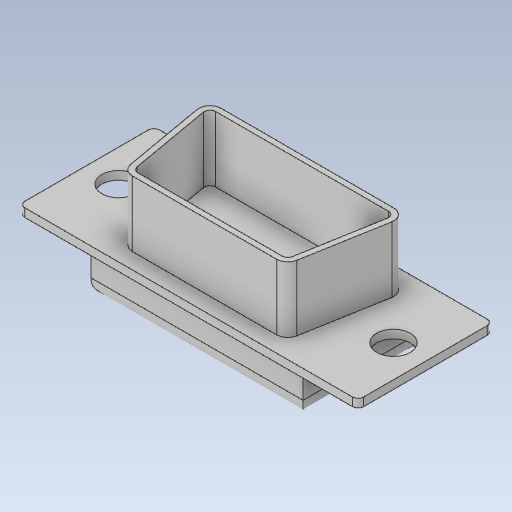
# Autodesk Inventor part: D-SUB
Saved by Autodesk Inventor 2020 (Build 240168000, 168)
## iProperties
Created: 2018-01-24
Part Number: D-SUB
Material: Generic
Document SubType Name: Modeling
Designer: Alex
Density: 1 g/cm^3
Appearance: Default
Author: Alex
Autodesk Inventor part; units mm, degrees
ref_plane "YZ Plane" through (0, 0, 0) normal (1, 0, 0) x (0, 1, 0)
ref_plane "XZ Plane" through (0, 0, 0) normal (0, 1, 0) x (-1, 0, 0)
ref_plane "XY Plane" through (0, 0, 0) normal (0, 0, 1) x (1, 0, 0)
sketch "Sketch1" plane through (0, 0, 0) normal (0, 1, 0) x (-1, 0, 0)
  line L0 (15.405, -6.125) -> (-15.405, -6.125)
  line L1 (-15.405, -6.125) -> (-15.405, 6.125)
  line L2 (-15.405, 6.125) -> (15.405, 6.125)
  line L3 (15.405, 6.125) -> (15.405, -6.125)
  line L4 (15.405, -6.125) -> (-15.405, 6.125) construction
  line L5 (-15.405, -6.125) -> (15.405, 6.125) construction
  point P0 (0, 0)
  point P1 (0, 0)
  dimension "d0" = 30.81
  dimension "d1" = 12.25
  constraints: 12 end point, 2 midpoint, 2 parallel, 1 coincident, 1 horizontal, 1 perpendicular
  measures "d0" distance of L1.end L2.end
  measures "d1" distance of L0.end L1.end
extrude "Extrusion1" add sketch "Sketch1" along normal blind 0.76
fillet "Fillet1" radius 0.5 4 edges at (15.405, 0.38, 6.125) (15.405, 0.38, -6.125) (-15.405, 0.38, 6.125) (-15.405, 0.38, -6.125)
sketch "Sketch2" plane through (0, 0.76, 0) normal (0, 1, 0) x (1, 0, 0)
  arc A0 (-14.905, 6.125) -> (-15.405, 5.625) centre (-14.905, 5.625) ccw construction
  line L0 (-15.405, 5.625) -> (-15.405, -5.625) construction
  arc A1 (-15.405, -5.625) -> (-14.905, -6.125) centre (-14.905, -5.625) ccw construction
  line L1 (-14.905, -6.125) -> (14.905, -6.125) construction
  arc A2 (14.905, -6.125) -> (15.405, -5.625) centre (14.905, -5.625) ccw construction
  line L2 (15.405, -5.625) -> (15.405, 5.625) construction
  arc A3 (15.405, 5.625) -> (14.905, 6.125) centre (14.905, 5.625) ccw construction
  line L3 (14.905, 6.125) -> (-14.905, 6.125) construction
  line L4 (-14.905, 6.125) -> (14.905, 6.125) construction
  line L5 (0, 6.125) -> (0, -6.125) construction
  line L6 (-14.905, -6.125) -> (14.905, -6.125) construction
  point P0 (0, 0)
  point P1 (-12.495, 0)
  point P2 (12.495, 0)
  point P3 (0, 0)
  dimension "d5" = 24.99
  constraints: 3 midpoint, 2 end point, 2 horizontal alignment, 1 symmetric about line
  measures "d5" distance of point (12.495, 0) point (-12.495, 0)
hole "Hole1" at (-12.495, 0.76, 0) at (12.495, 0.76, 0) direction (0, -1, 0) diameter 3.05 depth 8 tip angle 118
sketch "Sketch3" plane through (0, 0.76, 0) normal (0, 1, 0) x (1, 0, 0)
  line L0 (-7.8641, 4.18) -> (7.8641, 4.18)
  line L1 (8.3565, 3.5932) -> (7.0588, -3.7668)
  line L2 (6.5664, -4.18) -> (-6.5664, -4.18)
  line L3 (-7.0588, -3.7668) -> (-8.3565, 3.5932)
  line L4 (-14.905, 6.125) -> (14.905, 6.125) projected
  line L5 (0, 6.125) -> (0, -6.125) construction
  line L6 (-15.405, 0) -> (15.405, 0) construction
  line L7 (15.405, 5.625) -> (15.405, -5.625) projected
  circle A0 centre (-12.495, 0) radius 1.525 construction
  circle A1 centre (12.495, 0) radius 1.525 construction
  arc A2 (-14.905, 6.125) -> (-15.405, 5.625) centre (-14.905, 5.625) ccw construction
  line L8 (-15.405, 5.625) -> (-15.405, -5.625) construction
  arc A3 (-15.405, -5.625) -> (-14.905, -6.125) centre (-14.905, -5.625) ccw construction
  line L9 (-14.905, -6.125) -> (14.905, -6.125) construction
  arc A4 (14.905, -6.125) -> (15.405, -5.625) centre (14.905, -5.625) ccw construction
  line L10 (15.405, -5.625) -> (15.405, 5.625) construction
  arc A5 (15.405, 5.625) -> (14.905, 6.125) centre (14.905, 5.625) ccw construction
  line L11 (14.905, 6.125) -> (-14.905, 6.125) construction
  arc A6 (-7.8641, 4.18) -> (-8.3565, 3.5932) centre (-7.8641, 3.68) ccw
  arc A7 (-7.0588, -3.7668) -> (-6.5664, -4.18) centre (-6.5664, -3.68) ccw
  arc A8 (6.5664, -4.18) -> (7.0588, -3.7668) centre (6.5664, -3.68) ccw
  arc A9 (8.3565, 3.5932) -> (7.8641, 4.18) centre (7.8641, 3.68) ccw
  line L12 (7.8641, 4.68) -> (-7.8641, 4.68)
  arc A10 (-7.8641, 4.68) -> (-8.8489, 3.5064) centre (-7.8641, 3.68) ccw
  line L13 (-8.8489, 3.5064) -> (-7.5512, -3.8536)
  arc A11 (-7.5512, -3.8536) -> (-6.5664, -4.68) centre (-6.5664, -3.68) ccw
  line L14 (-6.5664, -4.68) -> (6.5664, -4.68)
  arc A12 (6.5664, -4.68) -> (7.5512, -3.8536) centre (6.5664, -3.68) ccw
  line L15 (7.5512, -3.8536) -> (8.8489, 3.5064)
  arc A13 (8.8489, 3.5064) -> (7.8641, 4.68) centre (7.8641, 3.68) ccw
  point P0 (0, 0)
  point P1 (-8.46, 4.18)
  point P2 (8.46, 4.18)
  dimension "d14" = 100
  dimension "d15" = 8.36
  dimension "d16" = 16.92
  dimension "d17" = 0.5
  dimension "d18" = 0.5
  constraints: 20 end point, 16 point on circle, 8 centre point, 8 tangent, 4 midpoint, 4 point on line, 3 equal radius, 2 parallel, 1 horizontal, 1 vertical, 9 other
  measures "d14" angle of L2 L3
  measures "d15" distance between parallel lines of L2 L0
  measures "d16" distance of point (-8.46, 4.18) point (8.46, 4.18)
  measures "d17" radius of A6
  measures "d18" distance between parallel lines of L0 L12
extrude "Extrusion2" add sketch "Sketch3" along normal blind 5.95
sketch "Sketch4" plane through (0, 0, 0) normal (0, -1, 0) x (1, 0, 0)
  circle A0 centre (-12.495, 0) radius 1.525 construction
  circle A1 centre (12.495, 0) radius 1.525 construction
  arc A2 (-15.405, -5.625) -> (-14.905, -6.125) centre (-14.905, -5.625) ccw construction
  line L0 (-14.905, -6.125) -> (14.905, -6.125) construction
  arc A3 (14.905, -6.125) -> (15.405, -5.625) centre (14.905, -5.625) ccw construction
  line L1 (15.405, -5.625) -> (15.405, 5.625) construction
  arc A4 (15.405, 5.625) -> (14.905, 6.125) centre (14.905, 5.625) ccw construction
  line L2 (14.905, 6.125) -> (-14.905, 6.125) construction
  arc A5 (-14.905, 6.125) -> (-15.405, 5.625) centre (-14.905, 5.625) ccw construction
  line L3 (-15.405, 5.625) -> (-15.405, -5.625) construction
  line L4 (0, -6.125) -> (0, 6.125) construction
  line L5 (-14.905, 6.125) -> (14.905, 6.125) construction
  line L6 (15.405, 5.625) -> (15.405, -5.625) construction
  line L7 (15.405, 0) -> (-15.405, 0) construction
  line L8 (-15.405, -5.625) -> (-15.405, 5.625) construction
  line L9 (-9.64, 5.36) -> (9.64, 5.36)
  line L10 (9.64, 5.36) -> (9.64, -5.36)
  line L11 (9.64, -5.36) -> (-9.64, -5.36)
  line L12 (-9.64, -5.36) -> (-9.64, 5.36)
  line L13 (-9.64, 5.36) -> (9.64, -5.36) construction
  line L14 (9.64, 5.36) -> (-9.64, -5.36) construction
  point P0 (0, 0)
  dimension "d21" = 19.28
  dimension "d22" = 10.72
  constraints: 16 end point, 6 midpoint, 2 parallel, 1 horizontal, 1 perpendicular
  measures "d21" distance of L10.end L11.end
  measures "d22" distance of L9.end L10.end
extrude "Extrusion3" add sketch "Sketch4" along normal blind 4.01
fillet "Fillet2" radius 1.5 4 edges at (0, -4.01, 5.36) (9.64, -4.01, 0) (-9.64, -4.01, 0) (0, -4.01, -5.36) curvature continuous yes
sketch "Sketch5" plane through (0, -4.01, 0) normal (0, -1, 0) x (1, 0, 0)
  line L0 (8.14, -3.86) -> (-8.14, -3.86) construction
  line L1 (8.14, 3.86) -> (8.14, -3.86) construction
  line L2 (-8.14, 3.86) -> (8.14, 3.86) construction
  line L3 (-8.14, -3.86) -> (-8.14, 3.86) construction
  line L4 (8.14, 3.86) -> (8.14, -3.86) construction
  line L5 (8.14, 0) -> (-8.14, 0) construction
  line L6 (-8.14, -3.86) -> (-8.14, 3.86) construction
  line L7 (8.14, -3.86) -> (-8.14, -3.86) construction
  line L8 (0, -3.86) -> (0, 3.86) construction
  line L9 (-8.14, 3.86) -> (8.14, 3.86) construction
  point P0 (0, 0)
  constraints: 4 end point, 4 midpoint
body "Solid1"
